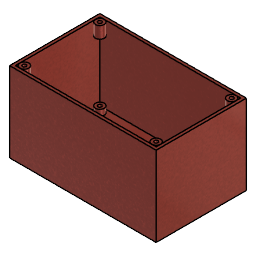
enclosure (Autodesk Fusion 360 design; units mm, degrees)
part number: 2026-09-24-22-09-04-954
Autodesk Fusion 360 part; units mm, degrees
sketch "BaseOuterProfile" plane through (0, 0, 0) normal (0, 0, 1) x (1, 0, 0)
  line L0 (0, 0) -> (99, 0)
  line L1 (99, 0) -> (99, 61)
  line L2 (99, 61) -> (0, 61)
  line L3 (0, 61) -> (0, 0)
extrude "Extrude1" add sketch "BaseOuterProfile" along normal blind 54 makes body 1
shell "Shell1" thickness 2 removed faces 1 at (33, 40.6667, 54) on bodies 1
ref_plane "WorkPlane1" through (0, 0, 2) normal (0, 0, 1) x (1, 0, 0)
sketch "StandoffPosts" plane through (0, 0, 2) normal (0, 0, 1) x (1, 0, 0)
  circle A0 centre (6, 6) radius 3
  circle A1 centre (93, 6) radius 3
  circle A2 centre (6, 55) radius 3
  circle A3 centre (93, 55) radius 3
extrude "Extrude2" add sketch "StandoffPosts" along normal blind 4 contours A0 bodies 1
extrude "Extrude3" add sketch "StandoffPosts" along normal blind 4 contours A2 bodies 1
extrude "Extrude4" add sketch "StandoffPosts" along normal blind 4 contours A1 bodies 1
extrude "Extrude5" add sketch "StandoffPosts" along normal blind 4 contours A3 bodies 1
sketch "StandoffPilotHoles" plane through (0, 0, 2) normal (0, 0, 1) x (1, 0, 0)
  circle A0 centre (6, 6) radius 1.25
  circle A1 centre (93, 6) radius 1.25
  circle A2 centre (6, 55) radius 1.25
  circle A3 centre (93, 55) radius 1.25
extrude "Extrude6" cut sketch "StandoffPilotHoles" along normal blind 4 contours A0 bodies 1
extrude "Extrude7" cut sketch "StandoffPilotHoles" along normal blind 4 contours A2 bodies 1
extrude "Extrude8" cut sketch "StandoffPilotHoles" along normal blind 4 contours A1 bodies 1
extrude "Extrude9" cut sketch "StandoffPilotHoles" along normal blind 4 contours A3 bodies 1
ref_plane "WorkPlane2" through (0, 0, 46) normal (0, 0, 1) x (1, 0, 0)
sketch "LidBossPosts" plane through (0, 0, 46) normal (0, 0, 1) x (1, 0, 0)
  circle A0 centre (5, 5) radius 3
  circle A1 centre (94, 5) radius 3
  circle A2 centre (5, 56) radius 3
  circle A3 centre (94, 56) radius 3
extrude "Extrude10" add sketch "LidBossPosts" along normal blind 8 contours A0 bodies 1
extrude "Extrude11" add sketch "LidBossPosts" along normal blind 8 contours A2 bodies 1
extrude "Extrude12" add sketch "LidBossPosts" along normal blind 8 contours A1 bodies 1
extrude "Extrude13" add sketch "LidBossPosts" along normal blind 8 contours A3 bodies 1
sketch "LidBossPilotHoles" plane through (0, 0, 46) normal (0, 0, 1) x (1, 0, 0)
  circle A0 centre (5, 5) radius 1.25
  circle A1 centre (94, 5) radius 1.25
  circle A2 centre (5, 56) radius 1.25
  circle A3 centre (94, 56) radius 1.25
extrude "Extrude14" cut sketch "LidBossPilotHoles" along normal blind 8 contours A0 bodies 1
extrude "Extrude15" cut sketch "LidBossPilotHoles" along normal blind 8 contours A2 bodies 1
extrude "Extrude16" cut sketch "LidBossPilotHoles" along normal blind 8 contours A1 bodies 1
extrude "Extrude17" cut sketch "LidBossPilotHoles" along normal blind 8 contours A3 bodies 1
ref_plane "WorkPlane3" through (0, 0, 54) normal (0, 0, 1) x (1, 0, 0)
sketch "LidOuterProfile" plane through (0, 0, 54) normal (0, 0, 1) x (1, 0, 0)
  line L0 (0, 0) -> (99, 0)
  line L1 (99, 0) -> (99, 61)
  line L2 (99, 61) -> (0, 61)
  line L3 (0, 61) -> (0, 0)
extrude "Extrude18" add sketch "LidOuterProfile" along normal blind 2 separate body makes body 2
sketch "LidClearanceHoles" plane through (0, 0, 54) normal (0, 0, 1) x (1, 0, 0)
  circle A0 centre (5, 5) radius 1.7
  circle A1 centre (94, 5) radius 1.7
  circle A2 centre (5, 56) radius 1.7
  circle A3 centre (94, 56) radius 1.7
extrude "Extrude19" cut sketch "LidClearanceHoles" along normal blind 2 contours A0 bodies 2
extrude "Extrude20" cut sketch "LidClearanceHoles" along normal blind 2 contours A2 bodies 2
extrude "Extrude21" cut sketch "LidClearanceHoles" along normal blind 2 contours A1 bodies 2
extrude "Extrude22" cut sketch "LidClearanceHoles" along normal blind 2 contours A3 bodies 2
hidden bodies 2
named bodies: "Enclosure_Base", "Enclosure_Lid"
